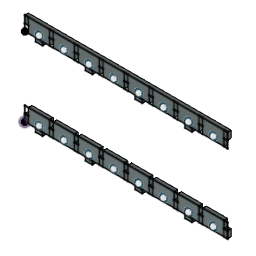
barre-échecs (Autodesk Fusion 360 design; units mm, degrees)
part number: 2026-06-29-15-08-07-008
Autodesk Fusion 360 part; units mm, degrees
sketch "Esquisse1" plane through (0, 0, 0) normal (0, 1, 0) x (1, 0, 0)
  line L0 (145, -20) -> (145, -10)
  line L1 (250, -20) -> (250, -10)
  line L2 (280, -10) -> (285, -10)
  line L3 (40, -20) -> (40, -10)
  line L4 (5, -10) -> (5, -20)
  line L5 (285, 0) -> (285, -20)
  line L6 (85, 0) -> (95, 0)
  line L7 (70, -10) -> (70, -20)
  line L8 (165, 0) -> (165, 5)
  line L9 (235, 0) -> (235, 5)
  line L10 (95, 5) -> (85, 5)
  line L11 (70, -20) -> (75, -20)
  line L12 (175, -10) -> (175, -20)
  line L13 (105, -10) -> (105, -20)
  line L14 (75, -20) -> (75, -10)
  line L15 (25, 5) -> (15, 5)
  line L16 (35, -20) -> (40, -20)
  line L17 (85, 5) -> (85, 0)
  line L18 (180, -20) -> (180, -10)
  line L19 (110, -20) -> (110, -10)
  line L20 (165, 5) -> (155, 5)
  line L21 (145, -10) -> (140, -10)
  line L22 (35, -10) -> (35, -20)
  line L23 (210, -10) -> (210, -20)
  line L24 (235, 5) -> (225, 5)
  line L25 (40, -10) -> (35, -10)
  line L26 (0, -20) -> (0, -10)
  line L27 (210, -20) -> (215, -20)
  line L28 (95, 0) -> (95, 5)
  line L29 (5, -20) -> (0, -20)
  line L30 (180, -10) -> (175, -10)
  line L31 (285, -10) -> (285, -20)
  line L32 (0, -20) -> (0, 0)
  line L33 (225, 5) -> (225, 0)
  line L34 (155, 0) -> (165, 0)
  line L35 (25, 0) -> (25, 5)
  line L36 (155, 5) -> (155, 0)
  line L37 (175, -20) -> (180, -20)
  line L38 (250, -10) -> (245, -10)
  line L39 (15, 5) -> (15, 0)
  line L40 (225, 0) -> (235, 0)
  line L41 (75, -10) -> (70, -10)
  line L42 (110, -10) -> (105, -10)
  line L43 (140, -20) -> (145, -20)
  line L44 (215, -10) -> (210, -10)
  line L45 (105, -20) -> (110, -20)
  line L46 (280, -20) -> (280, -10)
  line L47 (215, -20) -> (215, -10)
  line L48 (0, -10) -> (5, -10)
  line L49 (245, -10) -> (245, -20)
  line L50 (15, 0) -> (25, 0)
  line L51 (285, -20) -> (280, -20)
  line L52 (245, -20) -> (250, -20)
  line L53 (285, -20) -> (0, -20)
  line L54 (0, 0) -> (285, 0)
  line L55 (140, -10) -> (140, -20)
  line L56 (35, -10) -> (40, -10)
  line L57 (40, -10) -> (40, 0)
  line L58 (40, 0) -> (35, 0)
  line L59 (35, 0) -> (35, -10)
  line L60 (70, -10) -> (75, -10)
  line L61 (75, -10) -> (75, 0)
  line L62 (75, 0) -> (70, 0)
  line L63 (70, 0) -> (70, -10)
  line L64 (105, -10) -> (110, -10)
  line L65 (110, -10) -> (110, 0)
  line L66 (110, 0) -> (105, 0)
  line L67 (105, 0) -> (105, -10)
  line L68 (145, -10) -> (140, -10)
  line L69 (140, -10) -> (140, 0)
  line L70 (140, 0) -> (145, 0)
  line L71 (145, 0) -> (145, -10)
  line L72 (180, -10) -> (175, -10)
  line L73 (175, -10) -> (175, 0)
  line L74 (175, 0) -> (180, 0)
  line L75 (180, 0) -> (180, -10)
  line L76 (215, -10) -> (210, -10)
  line L77 (210, -10) -> (210, 0)
  line L78 (210, 0) -> (215, 0)
  line L79 (215, 0) -> (215, -10)
  line L80 (250, -10) -> (245, -10)
  line L81 (245, -10) -> (245, 0)
  line L82 (245, 0) -> (250, 0)
  line L83 (250, 0) -> (250, -10)
  line L84 (280, -10) -> (285, -10)
  line L85 (285, -10) -> (285, 0)
  line L86 (285, 0) -> (280, 0)
  line L87 (280, 0) -> (280, -10)
  line L88 (5, -10) -> (0, -10)
  line L89 (0, -10) -> (0, 0)
  line L90 (0, 0) -> (5, 0)
  line L91 (5, 0) -> (5, -10)
  line L92 (175, -110) -> (180, -110)
  line L93 (180, -120) -> (175, -120)
  line L94 (0, -110) -> (285, -110)
  line L95 (180, -120) -> (175, -120)
  line L96 (175, -130) -> (180, -130)
  line L97 (145, -130) -> (145, -120)
  line L98 (165, -105) -> (155, -105)
  line L99 (85, -110) -> (95, -110)
  line L100 (280, -120) -> (285, -120)
  line L101 (25, -105) -> (15, -105)
  line L102 (155, -105) -> (155, -110)
  line L103 (280, -130) -> (280, -120)
  line L104 (285, -110) -> (280, -110)
  line L105 (15, -105) -> (15, -110)
  line L106 (285, -110) -> (285, -130)
  line L107 (85, -105) -> (85, -110)
  line L108 (95, -105) -> (85, -105)
  line L109 (280, -120) -> (285, -120)
  line L110 (105, -110) -> (105, -120)
  line L111 (285, -120) -> (285, -110)
  line L112 (110, -130) -> (110, -120)
  line L113 (105, -120) -> (105, -130)
  line L114 (0, -130) -> (0, -120)
  line L115 (280, -110) -> (280, -120)
  line L116 (105, -130) -> (110, -130)
  line L117 (165, -110) -> (165, -105)
  line L118 (5, -110) -> (5, -120)
  line L119 (180, -110) -> (180, -120)
  line L120 (215, -120) -> (210, -120)
  line L121 (285, -130) -> (280, -130)
  line L122 (145, -120) -> (140, -120)
  line L123 (250, -130) -> (250, -120)
  line L124 (0, -120) -> (0, -110)
  line L125 (35, -110) -> (35, -120)
  line L126 (155, -110) -> (165, -110)
  line L127 (105, -120) -> (110, -120)
  line L128 (285, -120) -> (285, -130)
  line L129 (245, -120) -> (245, -110)
  line L130 (0, -130) -> (0, -110)
  line L131 (210, -110) -> (215, -110)
  line L132 (180, -130) -> (180, -120)
  line L133 (175, -120) -> (175, -110)
  line L134 (0, -120) -> (5, -120)
  line L135 (235, -105) -> (225, -105)
  line L136 (35, -130) -> (40, -130)
  line L137 (5, -120) -> (0, -120)
  line L138 (40, -120) -> (40, -110)
  line L139 (110, -120) -> (105, -120)
  line L140 (140, -120) -> (140, -110)
  line L141 (140, -110) -> (145, -110)
  line L142 (95, -110) -> (95, -105)
  line L143 (40, -110) -> (35, -110)
  line L144 (245, -120) -> (245, -130)
  line L145 (250, -120) -> (245, -120)
  line L146 (215, -130) -> (215, -120)
  line L147 (175, -120) -> (175, -130)
  line L148 (70, -120) -> (70, -130)
  line L149 (145, -120) -> (140, -120)
  line L150 (110, -120) -> (110, -110)
  line L151 (110, -110) -> (105, -110)
  line L152 (285, -130) -> (0, -130)
  line L153 (70, -110) -> (70, -120)
  line L154 (245, -110) -> (250, -110)
  line L155 (15, -110) -> (25, -110)
  line L156 (35, -120) -> (40, -120)
  line L157 (215, -110) -> (215, -120)
  line L158 (250, -120) -> (245, -120)
  line L159 (210, -120) -> (210, -110)
  line L160 (75, -130) -> (75, -120)
  line L161 (210, -130) -> (215, -130)
  line L162 (40, -120) -> (35, -120)
  line L163 (235, -110) -> (235, -105)
  line L164 (225, -105) -> (225, -110)
  line L165 (140, -120) -> (140, -130)
  line L166 (5, -130) -> (0, -130)
  line L167 (75, -120) -> (70, -120)
  line L168 (35, -120) -> (35, -130)
  line L169 (215, -120) -> (210, -120)
  line L170 (40, -130) -> (40, -120)
  line L171 (0, -110) -> (5, -110)
  line L172 (70, -120) -> (75, -120)
  line L173 (5, -120) -> (5, -130)
  line L174 (145, -110) -> (145, -120)
  line L175 (210, -120) -> (210, -130)
  line L176 (25, -110) -> (25, -105)
  line L177 (140, -130) -> (145, -130)
  line L178 (70, -130) -> (75, -130)
  line L179 (75, -110) -> (70, -110)
  line L180 (225, -110) -> (235, -110)
  line L181 (75, -120) -> (75, -110)
  line L182 (250, -110) -> (250, -120)
  line L183 (245, -130) -> (250, -130)
  circle A0 centre (20, -5) radius 5
  circle A1 centre (55, -5) radius 5
  circle A2 centre (90, -5) radius 5
  circle A3 centre (125, -5) radius 5
  circle A4 centre (160, -5) radius 5
  circle A5 centre (195, -5) radius 5
  circle A6 centre (230, -5) radius 5
  circle A7 centre (265, -5) radius 5
  circle A8 centre (20, -115) radius 5
  circle A9 centre (55, -115) radius 5
  circle A10 centre (90, -115) radius 5
  circle A11 centre (125, -115) radius 5
  circle A12 centre (160, -115) radius 5
  circle A13 centre (195, -115) radius 5
  circle A14 centre (230, -115) radius 5
  circle A15 centre (265, -115) radius 5
  point P0 (0, -110)
  point P1 (0, -110)
  dimension "d38" = 15
  dimension "d39" = 10
  dimension "d40" = 60
  dimension "d41" = 60
  dimension "d42" = 60
  dimension "d43" = 50
  dimension "d44" = 5
  dimension "d45" = 20
  dimension "d46" = 5
  dimension "d47" = 10
  dimension "d48" = 10
  dimension "d49" = 10
  dimension "d50" = 10
  dimension "d51" = 10
  dimension "d52" = 10
  dimension "d53" = 10
  dimension "d54" = 10
  dimension "d57" = 15
  dimension "d58" = 10
  dimension "d59" = 60
  dimension "d60" = 60
  dimension "d61" = 60
  dimension "d62" = 50
  dimension "d63" = 5
  dimension "d64" = 20
  dimension "d65" = 5
  dimension "d66" = 10
  dimension "d67" = 10
  dimension "d68" = 10
  dimension "d69" = 10
  dimension "d70" = 10
  dimension "d71" = 10
  dimension "d72" = 10
  dimension "d73" = 10
  dimension "d76" = 35
  dimension "d77" = -110
  dimension "d80" = 110
  constraint horizontal L54
  constraint vertical L5
  constraint horizontal L53
  constraint vertical L32
  constraint coincident L32.end L54.start
  constraint horizontal L50
  constraint vertical L35
  constraint horizontal L15
  constraint vertical L39
  constraint coincident L39.end L54
  constraint horizontal L6
  constraint vertical L28
  constraint horizontal L10
  constraint vertical L17
  constraint coincident L6.start L54
  constraint horizontal L34
  constraint vertical L8
  constraint horizontal L20
  constraint vertical L36
  constraint coincident L34.start L54
  constraint horizontal L40
  constraint vertical L9
  constraint horizontal L24
  constraint vertical L33
  constraint coincident L33.end L54
  constraint equal L10 L15
  constraint equal L20 L24
  constraint equal L10 L20
  constraint collinear L10 L15
  constraint collinear L10 L20
  constraint collinear L20 L24
  constraint horizontal L16
  constraint vertical L3
  constraint horizontal L25
  constraint vertical L22
  constraint coincident L16.start L53
  constraint horizontal L11
  constraint vertical L14
  constraint horizontal L41
  constraint vertical L7
  constraint coincident L7.end L53
  constraint horizontal L45
  constraint vertical L19
  constraint horizontal L42
  constraint vertical L13
  constraint coincident L13.end L53
  constraint horizontal L43
  constraint vertical L0
  constraint horizontal L21
  constraint vertical L55
  constraint coincident L43.start L53
  constraint horizontal L37
  constraint vertical L18
  constraint horizontal L30
  constraint vertical L12
  constraint coincident L12.end L53
  constraint horizontal L27
  constraint vertical L47
  constraint horizontal L44
  constraint vertical L23
  constraint coincident L23.end L53
  constraint horizontal L52
  constraint vertical L1
  constraint horizontal L38
  constraint vertical L49
  constraint coincident L49.end L53
  constraint equal L25 L41
  constraint equal L41 L42
  constraint equal L21 L42
  constraint equal L21 L30
  constraint equal L30 L44
  constraint equal L38 L44
  constraint horizontal L29
  constraint vertical L26
  constraint horizontal L48
  constraint vertical L4
  constraint coincident L26.end L32
  constraint coincident L4.end L53
  constraint equal L3 L4
  constraint equal L25 L48
  constraint horizontal L51
  constraint vertical L46
  constraint horizontal L2
  constraint vertical L31
  constraint equal L2 L38
  constraint equal L1 L46
  constraint equal L47 L49
  constraint equal L18 L23
  constraint equal L0 L12
  constraint equal L19 L55
  constraint equal L13 L14
  constraint equal L3 L7
  constraint horizontal L56
  constraint vertical L57
  constraint horizontal L58
  constraint vertical L59
  constraint coincident L54 L57.end
  constraint horizontal L60
  constraint vertical L61
  constraint horizontal L62
  constraint vertical L63
  constraint coincident L54 L61.end
  constraint horizontal L64
  constraint vertical L65
  constraint horizontal L66
  constraint vertical L67
  constraint coincident L54 L65.end
  constraint horizontal L68
  constraint vertical L69
  constraint horizontal L70
  constraint vertical L71
  constraint coincident L54 L69.end
  constraint horizontal L72
  constraint vertical L73
  constraint horizontal L74
  constraint vertical L75
  constraint coincident L54 L73.end
  constraint horizontal L76
  constraint vertical L77
  constraint horizontal L78
  constraint vertical L79
  constraint coincident L54 L77.end
  constraint horizontal L80
  constraint vertical L81
  constraint horizontal L82
  constraint vertical L83
  constraint coincident L54 L81.end
  constraint horizontal L84
  constraint vertical L85
  constraint horizontal L86
  constraint vertical L87
  constraint horizontal L88
  constraint vertical L89
  constraint horizontal L90
  constraint vertical L91
  constraint collinear L3 L57
  constraint collinear L14 L61
  constraint collinear L19 L65
  constraint collinear L55 L69
  constraint collinear L12 L73
  constraint collinear L23 L77
  constraint collinear L49 L81
  constraint horizontal L94
  constraint vertical L106
  constraint horizontal L152
  constraint vertical L130
  constraint coincident P1 P0
  constraint horizontal L155
  constraint vertical L176
  constraint horizontal L101
  constraint vertical L105
  constraint coincident L105.end L94
  constraint horizontal L99
  constraint vertical L142
  constraint horizontal L108
  constraint vertical L107
  constraint coincident L99.start L94
  constraint horizontal L126
  constraint vertical L117
  constraint horizontal L98
  constraint vertical L102
  constraint coincident L102.end L94
  constraint horizontal L180
  constraint vertical L163
  constraint horizontal L135
  constraint vertical L164
  constraint coincident L164.end L94
  constraint equal L101 L108
  constraint equal L98 L135
  constraint equal L98 L108
  constraint collinear L101 L108
  constraint collinear L98 L108
  constraint collinear L98 L135
  constraint horizontal L136
  constraint vertical L170
  constraint horizontal L162
  constraint vertical L168
  constraint coincident L136.start L152
  constraint horizontal L178
  constraint vertical L160
  constraint horizontal L167
  constraint vertical L148
  constraint coincident L148.end L152
  constraint horizontal L116
  constraint vertical L112
  constraint horizontal L139
  constraint vertical L113
  constraint coincident L113.end L152
  constraint horizontal L177
  constraint vertical L97
  constraint horizontal L122
  constraint vertical L165
  constraint coincident L165.end L152
  constraint horizontal L96
  constraint vertical L132
  constraint horizontal L95
  constraint vertical L147
  constraint coincident L96.start L152
  constraint horizontal L161
  constraint vertical L146
  constraint horizontal L120
  constraint vertical L175
  constraint coincident L161.start L152
  constraint horizontal L183
  constraint vertical L123
  constraint horizontal L158
  constraint vertical L144
  constraint coincident L144.end L152
  constraint equal L162 L167
  constraint equal L139 L167
  constraint equal L122 L139
  constraint equal L95 L122
  constraint equal L95 L120
  constraint equal L120 L158
  constraint horizontal L166
  constraint vertical L114
  constraint horizontal L134
  constraint vertical L173
  constraint coincident L114.end L130
  constraint coincident L166.start L152
  constraint equal L170 L173
  constraint equal L134 L162
  constraint horizontal L121
  constraint vertical L103
  constraint horizontal L109
  constraint vertical L128
  constraint equal L109 L158
  constraint equal L103 L123
  constraint equal L144 L146
  constraint equal L132 L175
  constraint equal L97 L147
  constraint equal L112 L165
  constraint equal L113 L160
  constraint equal L148 L170
  constraint horizontal L156
  constraint vertical L138
  constraint horizontal L143
  constraint vertical L125
  constraint coincident L138.end L94
  constraint horizontal L172
  constraint vertical L181
  constraint horizontal L179
  constraint vertical L153
  constraint coincident L179.start L94
  constraint horizontal L127
  constraint vertical L150
  constraint horizontal L151
  constraint vertical L110
  constraint coincident L150.end L94
  constraint horizontal L149
  constraint vertical L140
  constraint horizontal L141
  constraint vertical L174
  constraint coincident L140.end L94
  constraint horizontal L93
  constraint vertical L133
  constraint horizontal L92
  constraint vertical L119
  constraint coincident L92.start L94
  constraint horizontal L169
  constraint vertical L159
  constraint horizontal L131
  constraint vertical L157
  constraint coincident L131.start L94
  constraint horizontal L145
  constraint vertical L129
  constraint horizontal L154
  constraint vertical L182
  constraint coincident L129.end L94
  constraint horizontal L100
  constraint vertical L111
  constraint horizontal L104
  constraint vertical L115
  constraint horizontal L137
  constraint vertical L124
  constraint horizontal L171
  constraint vertical L118
  constraint collinear L138 L170
  constraint collinear L160 L181
  constraint collinear L112 L150
  constraint collinear L140 L165
  constraint collinear L133 L147
  constraint collinear L159 L175
  constraint collinear L129 L144
  measures "d38" distance of L32.end L39
  measures "d39" distance of L15.start L15.end
  measures "d40" distance of L17 L35
  measures "d41" distance of L28 L36
  measures "d42" distance of L8 L33
  measures "d43" distance of L9.start L5
  measures "d44" distance of L15.end L39.end
  measures "d45" distance of L32.end L26.start
  measures "d46" distance of L3.end L22.start
  measures "d47" distance of L16.start L22.start
  measures "d48" distance of L22 L35
  measures "d49" distance of L14 L17
  measures "d50" distance of L13 L28
  measures "d51" distance of L0 L36
  measures "d52" distance of L8 L12
  measures "d53" distance of L33 L47
  measures "d54" distance of L9 L49
  measures "d57" distance of P1 L105
  measures "d58" distance of L101.start L101.end
  measures "d59" distance of L107 L176
  measures "d60" distance of L102 L142
  measures "d61" distance of L117 L164
  measures "d62" distance of L163.start L106
  measures "d63" distance of L105.end L101.end
  measures "d64" distance of L114.start P1
  measures "d65" distance of L125.end L138.start
  measures "d66" distance of L125.end L136.start
  measures "d67" distance of L168 L176
  measures "d68" distance of L107 L160
  measures "d69" distance of L113 L142
  measures "d70" distance of L97 L102
  measures "d71" distance of L117 L147
  measures "d72" distance of L146 L164
  measures "d73" distance of L144 L163
  measures "d80" distance of L32.end P1
extrude "Extrusion3" add sketch "Esquisse1" along normal blind 5 contours L0 L12 L34 L53 L54 L71 L73 | L21 L54 L68 L69 L70 L71 | A3 | L19 L53 L54 L55 L65 L69 | L30 L54 L72 L73 L74 L75 | A5 | L18 L23 L53 L54 L75 L77 | L8 L20 L34 L36 L54 | L42 L54 L64 L65 L66 L67 | L6 L13 L14 L53 L54 L61 L67 | L44 L54 L76 L77 L78 L79 | L40 L47 L49 L53 L54 L79 L81 | A1 | L3 L7 L53 L54 L57 L63 | L41 L54 L60 L61 L62 L63 | L6 L10 L17 L28 L54 | L38 L54 L80 L81 L82 L83 | A7 | L1 L46 L53 L54 L83 L87 | L25 L54 L56 L57 L58 L59 | L4 L22 L50 L53 L54 L59 L91 | L9 L24 L33 L40 L54 | L2 L5 L54 L84 L85 L86 L87 | L32 L48 L54 L88 L89 L90 L91 | L15 L35 L39 L50 L54 | L94 L97 L126 L133 L147 L152 L174 | A13 | L94 L119 L132 L152 L159 L175 | L94 L98 L102 L117 L126 | L93 L95 L96 L132 L147 L152 | L97 L122 L149 L152 L165 L177 | L94 L129 L144 L146 L152 L157 L180 | L120 L146 L152 L161 L169 L175 | A11 | L94 L112 L140 L150 L152 L165 | L94 L135 L163 L164 L180 | L112 L113 L116 L127 L139 L152 | L123 L144 L145 L152 L158 L183 | L94 L99 L110 L113 L152 L160 L181 | A15 | L94 L103 L115 L123 L152 L182 | L148 L152 L160 L167 L172 L178 | L100 L103 L106 L109 L121 L128 L152 | A9 | L94 L138 L148 L152 L153 L170 | L94 L99 L107 L108 L142 | L136 L152 L156 L162 L168 L170 | L94 L118 L125 L152 L155 L168 L173 | L114 L130 L134 L137 L152 L166 L173 | L94 L101 L105 L155 L176 makes body 1 at (188.3333, 0, 3.3333) makes body 2 at (141.6667, 5, 126.6667)
extrude "Extrusion4" cut sketch "Esquisse1" along normal blind 15 contours A3 | A5 | A1 | A7 | A13 | A11 | A15 | A9 bodies 1 2
sketch "Esquisse2" plane through (0, 5, 0) normal (0, 1, 0) x (-1, 0, 0)
  line L0 (0, 130) -> (-285, 130)
  line L1 (-285, 130) -> (-285, 120)
  line L2 (-285, 120) -> (-280, 120)
  line L3 (-280, 120) -> (-280, 110)
  line L4 (-280, 110) -> (-265, 110)
  circle A0 centre (-265, 115) radius 5
  line L5 (-265, 110) -> (-250, 110)
  line L6 (-250, 110) -> (-250, 120)
  line L7 (-250, 120) -> (-245, 120)
  line L8 (-245, 120) -> (-245, 110)
  line L9 (-245, 110) -> (-235, 110)
  line L10 (-235, 110) -> (-235, 105)
  line L11 (-235, 105) -> (-225, 105)
  line L12 (-225, 105) -> (-225, 110)
  line L13 (-225, 110) -> (-215, 110)
  line L14 (-215, 110) -> (-215, 120)
  line L15 (-215, 120) -> (-210, 120)
  line L16 (-210, 120) -> (-210, 110)
  line L17 (-210, 110) -> (-195, 110)
  circle A1 centre (-195, 115) radius 5
  line L18 (-195, 110) -> (-180, 110)
  line L19 (-180, 110) -> (-180, 120)
  line L20 (-180, 120) -> (-175, 120)
  line L21 (-175, 120) -> (-175, 110)
  line L22 (-175, 110) -> (-165, 110)
  line L23 (-165, 110) -> (-165, 105)
  line L24 (-165, 105) -> (-155, 105)
  line L25 (-155, 105) -> (-155, 110)
  line L26 (-155, 110) -> (-145, 110)
  line L27 (-145, 110) -> (-145, 120)
  line L28 (-145, 120) -> (-140, 120)
  line L29 (-140, 120) -> (-140, 110)
  line L30 (-140, 110) -> (-125, 110)
  circle A2 centre (-125, 115) radius 5
  line L31 (-125, 110) -> (-110, 110)
  line L32 (-110, 110) -> (-110, 120)
  line L33 (-110, 120) -> (-105, 120)
  line L34 (-105, 120) -> (-105, 110)
  line L35 (-105, 110) -> (-95, 110)
  line L36 (-95, 110) -> (-95, 105)
  line L37 (-95, 105) -> (-85, 105)
  line L38 (-85, 105) -> (-85, 110)
  line L39 (-85, 110) -> (-75, 110)
  line L40 (-75, 110) -> (-75, 120)
  line L41 (-75, 120) -> (-70, 120)
  line L42 (-70, 120) -> (-70, 110)
  line L43 (-70, 110) -> (-55, 110)
  circle A3 centre (-55, 115) radius 5
  line L44 (-55, 110) -> (-40, 110)
  line L45 (-40, 110) -> (-40, 120)
  line L46 (-40, 120) -> (-35, 120)
  line L47 (-35, 120) -> (-35, 110)
  line L48 (-35, 110) -> (-25, 110)
  line L49 (-25, 110) -> (-25, 105)
  line L50 (-25, 105) -> (-15, 105)
  line L51 (-15, 105) -> (-15, 110)
  line L52 (-15, 110) -> (-5, 110)
  line L53 (-5, 110) -> (-5, 120)
  line L54 (-5, 120) -> (0, 120)
  line L55 (0, 120) -> (0, 130)
  circle A4 centre (-20, 115) radius 5
  circle A5 centre (-90, 115) radius 5
  circle A6 centre (-160, 115) radius 5
  circle A7 centre (-230, 115) radius 5
sketch "Esquisse3" plane through (0, 5, 0) normal (0, 1, 0) x (-1, 0, 0)
  line L0 (-85, 0) -> (-55, 0)
  circle A0 centre (-55, 5) radius 5
  line L1 (-55, 0) -> (-25, 0)
  line L2 (-25, 0) -> (-25, -5)
  line L3 (-25, -5) -> (-15, -5)
  line L4 (-15, -5) -> (-15, 0)
  line L5 (-15, 0) -> (0, 0)
  line L6 (0, 0) -> (0, 10)
  line L7 (0, 10) -> (-5, 10)
  line L8 (-5, 10) -> (-5, 20)
  line L9 (-5, 20) -> (-35, 20)
  line L10 (-35, 20) -> (-35, 10)
  line L11 (-35, 10) -> (-40, 10)
  line L12 (-40, 10) -> (-40, 20)
  line L13 (-40, 20) -> (-70, 20)
  line L14 (-70, 20) -> (-70, 10)
  line L15 (-70, 10) -> (-75, 10)
  line L16 (-75, 10) -> (-75, 20)
  line L17 (-75, 20) -> (-105, 20)
  line L18 (-105, 20) -> (-105, 10)
  line L19 (-105, 10) -> (-110, 10)
  line L20 (-110, 10) -> (-110, 20)
  line L21 (-110, 20) -> (-140, 20)
  line L22 (-140, 20) -> (-140, 10)
  line L23 (-140, 10) -> (-145, 10)
  line L24 (-145, 10) -> (-145, 20)
  line L25 (-145, 20) -> (-175, 20)
  line L26 (-175, 20) -> (-175, 10)
  line L27 (-175, 10) -> (-180, 10)
  line L28 (-180, 10) -> (-180, 20)
  line L29 (-180, 20) -> (-210, 20)
  line L30 (-210, 20) -> (-210, 10)
  line L31 (-210, 10) -> (-215, 10)
  line L32 (-215, 10) -> (-215, 20)
  line L33 (-215, 20) -> (-245, 20)
  line L34 (-245, 20) -> (-245, 10)
  line L35 (-245, 10) -> (-250, 10)
  line L36 (-250, 10) -> (-250, 20)
  line L37 (-250, 20) -> (-280, 20)
  line L38 (-280, 20) -> (-280, 10)
  line L39 (-280, 10) -> (-285, 10)
  line L40 (-285, 10) -> (-285, 0)
  line L41 (-285, 0) -> (-265, 0)
  circle A1 centre (-265, 5) radius 5
  line L42 (-265, 0) -> (-235, 0)
  line L43 (-235, 0) -> (-235, -5)
  line L44 (-235, -5) -> (-225, -5)
  line L45 (-225, -5) -> (-225, 0)
  line L46 (-225, 0) -> (-195, 0)
  circle A2 centre (-195, 5) radius 5
  line L47 (-195, 0) -> (-165, 0)
  line L48 (-165, 0) -> (-165, -5)
  line L49 (-165, -5) -> (-155, -5)
  line L50 (-155, -5) -> (-155, 0)
  line L51 (-155, 0) -> (-125, 0)
  circle A3 centre (-125, 5) radius 5
  line L52 (-125, 0) -> (-95, 0)
  line L53 (-95, 0) -> (-95, -5)
  line L54 (-95, -5) -> (-85, -5)
  line L55 (-85, -5) -> (-85, 0)
  circle A4 centre (-230, 5) radius 5
  circle A5 centre (-20, 5) radius 5
  circle A6 centre (-160, 5) radius 5
  circle A7 centre (-90, 5) radius 5
